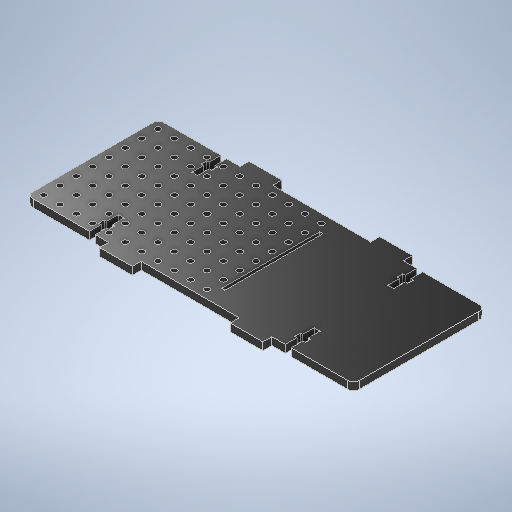
# Autodesk Inventor part: Mounting Base Middle
Saved by Autodesk Inventor 2025.1 (Build 291241000, 241)
## iProperties
Created: 2024-05-30
Part Number: Mounting Base Middle
Material: Polycarbonate, Smoke
Document SubType Name: Modeling
Designer: AlexForbes
Density: 1.2 g/cm^3
Appearance: Glossy - Black
Author: AlexForbes
Autodesk Inventor part; units mm, degrees
ref_plane "YZ Plane" through (0, 0, 0) normal (1, 0, 0) x (0, 1, 0)
ref_plane "XZ Plane" through (0, 0, 0) normal (0, 1, 0) x (-1, 0, 0)
sketch "Sketch1" plane through (0, 0, 0) normal (0, 1, 0) x (-1, 0, 0)
  line L0 (0, 0) -> (-254, 0)
  line L1 (-254, 0) -> (-254, -102.3)
  line L2 (-254, -102.3) -> (0, -102.3)
  line L3 (0, -102.3) -> (0, 0)
  dimension "d19" = 102.3
  dimension "d31" = 254
  constraints: 8 end point, 2 parallel, 1 horizontal, 1 perpendicular
  measures "d19" distance of L0.end L1.end
  measures "d31" distance of L1.end L2.end
extrude "Extrusion1" add sketch "Sketch1" along normal blind 6
ref_plane "Work Plane1" through (254, 0, -51.15) normal (0, 0, -1) x (-1, 0, 0)
sketch "Sketch3" plane through (0, 0, 0) normal (0, 1, 0) x (-1, 0, 0)
  line L0 (0, -102.3) -> (0, 0) projected
  line L1 (0, 0) -> (-254, 0) projected
  line L2 (-254, 0) -> (-254, -102.3) projected
  line L3 (-254, -102.3) -> (0, -102.3) projected
  line L4 (-63.5, -102.3) -> (-88.9, -102.3)
  line L5 (-88.9, -102.3) -> (-88.9, -109.3)
  line L6 (-88.9, -109.3) -> (-63.5, -109.3)
  line L7 (-63.5, -109.3) -> (-63.5, -102.3)
  line L8 (-165.1, -102.3) -> (-190.5, -102.3)
  line L9 (-190.5, -102.3) -> (-190.5, -109.3)
  line L10 (-190.5, -109.3) -> (-165.1, -109.3)
  line L11 (-165.1, -109.3) -> (-165.1, -102.3)
  line L12 (-88.9, -109.3) -> (-165.1, -109.3) construction
  point P0 (-127, -109.3)
  point P1 (-127, -102.3)
  point P2 (-88.9, -102.3)
  point P3 (-165.1, -102.3)
  point P4 (-190.5, -102.3)
  dimension "d20" = 7
  dimension "d21" = 76.2
  dimension "d32" = 25.4
  constraints: 18 end point, 4 parallel, 3 horizontal, 2 midpoint, 2 perpendicular, 2 point on line, 1 collinear, 1 horizontal alignment, 1 vertical alignment
  measures "d20" distance of L4.end L5.end
  measures "d21" distance of L5.end L10.end
  measures "d32" distance of L9.end L10.end
extrude "Extrusion2" add sketch "Sketch3" along normal up to surface (6 mm away) contours L7 L6 L5 L3 | L11 L10 L9 L3
mirror "Mirror1" about plane through (254, 0, -51.15) normal (0, 0, -1) of "Extrusion2"
sketch "Sketch4" plane through (0, 6, 0) normal (0, 1, 0) x (1, 0, 0)
  line L0 (124.7521, 22.5) -> (129.2479, 22.5) construction
  line L1 (122.875, 13.375) -> (122.875, 9.125) construction
  line L2 (131.125, 9.125) -> (131.125, 13.375) construction
  line L3 (124.7521, 0) -> (124.7521, 9.125) construction
  line L4 (124.7521, 13.375) -> (124.7521, 22.5) construction
  line L5 (129.2479, 22.5) -> (129.2479, 13.375) construction
  line L6 (129.2479, 9.125) -> (129.2479, 0) construction
  line L7 (131.125, 13.375) -> (129.2479, 13.375) construction
  line L8 (124.7521, 13.375) -> (122.875, 13.375) construction
  line L9 (122.875, 9.125) -> (124.7521, 9.125) construction
  line L10 (129.2479, 9.125) -> (131.125, 9.125) construction
  line L11 (124.7521, 0) -> (129.2479, 0) construction
  line L12 (88.9, 0) -> (165.1, 0) projected
  line L13 (48.5521, 22.5) -> (53.0479, 22.5)
  line L14 (48.5521, 13.375) -> (48.5521, 22.5)
  line L15 (46.675, 13.375) -> (46.675, 9.125)
  line L16 (48.5521, 0) -> (48.5521, 9.125)
  line L17 (54.925, 9.125) -> (54.925, 13.375)
  line L18 (46.675, 9.125) -> (48.5521, 9.125)
  line L19 (48.5521, 13.375) -> (46.675, 13.375)
  line L20 (53.0479, 9.125) -> (53.0479, 0)
  line L21 (53.0479, 22.5) -> (53.0479, 13.375)
  line L22 (54.925, 13.375) -> (53.0479, 13.375)
  line L23 (53.0479, 9.125) -> (54.925, 9.125)
  line L24 (48.5521, 0) -> (53.0479, 0)
  line L25 (200.9521, 22.5) -> (205.4479, 22.5)
  line L26 (200.9521, 13.375) -> (200.9521, 22.5)
  line L27 (199.075, 13.375) -> (199.075, 9.125)
  line L28 (200.9521, 0) -> (200.9521, 9.125)
  line L29 (207.325, 9.125) -> (207.325, 13.375)
  line L30 (199.075, 9.125) -> (200.9521, 9.125)
  line L31 (200.9521, 13.375) -> (199.075, 13.375)
  line L32 (205.4479, 9.125) -> (205.4479, 0)
  line L33 (205.4479, 22.5) -> (205.4479, 13.375)
  line L34 (207.325, 13.375) -> (205.4479, 13.375)
  line L35 (205.4479, 9.125) -> (207.325, 9.125)
  line L36 (200.9521, 0) -> (205.4479, 0)
  point P0 (0, 0)
  point P1 (127, 22.5)
  point P2 (127, 0)
  point P3 (50.8, 22.5)
  point P4 (50.8, 0)
  point P5 (203.2, 22.5)
  point P6 (203.2, 0)
  point P7 (127, 0)
  point P8 (127, 0)
  point P9 (127, 0)
  point P10 (127, 0)
  dimension "d24" = 22.5
  dimension "d25" = 4.25
  dimension "d26" = 8.25
  dimension "d28" = 4.4958
  dimension "d43" = 76.2
  dimension "d44" = 76.2
  constraints: 72 end point, 27 parallel, 20 equal length, 12 perpendicular, 11 midpoint, 8 horizontal alignment, 6 vertical, 3 horizontal, 3 vertical alignment
  measures "d24" distance of L0.end L6.end
  measures "d25" distance of L2.end L2.start
  measures "d26" distance of L2.start L1.end
  measures "d28" distance between parallel lines of L5 L4
  measures "d43" distance of point (127, 0) point (50.8, 0)
  measures "d44" distance of point (127, 0) point (203.2, 0)
extrude "Extrusion3" cut sketch "Sketch4" against normal through all
fillet "Fillet1" radius 5 4 edges at (0, 3, 0) (254, 3, 0) (254, 3, -102.3) (0, 3, -102.3) curvature continuous yes
mirror "Mirror2" about plane through (254, 0, -51.15) normal (0, 0, -1) of "Extrusion3"
sketch "Sketch2" plane through (0, 6, 0) normal (0, 1, 0) x (1, 0, 0)
  line L0 (0, 0) -> (0, 6.7) construction
  line L1 (0, 6.7) -> (6.35, 6.7) construction
  line L2 (6.35, 6.7) -> (6.35, 0) construction
  line L3 (6.35, 0) -> (0, 0) construction
  dimension "d3" = 6.7
  dimension "d45" = 6.35
  constraints: 8 end point, 2 parallel, 1 coincident, 1 perpendicular, 1 vertical
  measures "d3" distance of L1.end L2.end
  measures "d45" distance of L0.end L1.end
hole "Hole1" at (6.35, 6, -6.7) direction (0, -1, 0) diameter 4.25 end through all
pattern_linear "Rectangular Pattern1" count 11 spacing 12.7 along (1, 0, 0) count 8 spacing 12.7 along (0, 0, -1) of "Hole1"
sketch "Sketch6" plane through (0, 6, 0) normal (0, 1, 0) x (1, 0, 0)
  line L0 (138.43, 89.25) -> (140.97, 89.25)
  line L1 (140.97, 89.25) -> (140.97, 13.05)
  line L2 (140.97, 13.05) -> (138.43, 13.05)
  line L3 (138.43, 13.05) -> (138.43, 89.25)
  line L4 (0, 97.3) -> (0, 5) construction
  circle A0 centre (133.35, 95.6) radius 2.125 construction
  point P0 (0, 0)
  point P1 (138.43, 51.15)
  point P2 (0, 51.15)
  point P3 (139.7, 89.25)
  dimension "d50" = 2.54
  dimension "d51" = 76.2
  dimension "d53" = 139.7
  constraints: 8 end point, 3 midpoint, 2 parallel, 1 horizontal, 1 horizontal alignment, 1 perpendicular
  measures "d50" distance between parallel lines of L1 L3
  measures "d51" distance of L0.end L1.end
  measures "d53" distance from line of L4 point (139.7, 89.25)
extrude "Extrusion5" cut sketch "Sketch6" against normal blind 2.54
sketch "Sketch7" plane through (0, 0, 0) normal (0, -1, 0) x (1, 0, 0)
  point P0 (82.55, -57.5)
hole "Hole2" at (82.55, 0, -57.5) direction (0, 1, 0) diameter 4.5 end through all
body "Solid1"
